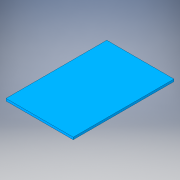
# Autodesk Inventor part: CBBLeft2
Saved by Autodesk Inventor 2019 (Build 230136000, 136)
## iProperties
Created: 2019-02-21
Part Number: CBBLeft2
Material: Generic
Document SubType Name: Modeling
Designer: james
Density: 1 g/cm^3
Appearance: Default(3)
Author: james
Autodesk Inventor part; units mm, degrees
ref_plane "YZ Plane" through (0, 0, 0) normal (1, 0, 0) x (0, 1, 0)
ref_plane "XZ Plane" through (0, 0, 0) normal (0, 1, 0) x (-1, 0, 0)
ref_plane "XY Plane" through (0, 0, 0) normal (0, 0, 1) x (1, 0, 0)
sketch "Sketch1" plane through (0, 0, 0) normal (0, 1, 0) x (-1, 0, 0)
  line L0 (59.2048, 125.73) -> (-93.1952, 125.73)
  line L1 (-93.1952, 125.73) -> (-93.1952, -102.87)
  line L2 (-93.1952, -102.87) -> (59.2048, -102.87)
  line L3 (59.2048, -102.87) -> (59.2048, 125.73)
  point P0 (0, 0)
  dimension "d0" = 228.6
  dimension "d1" = 152.4
  constraints: 8 end point, 2 parallel, 1 horizontal, 1 perpendicular
  measures "d0" distance of L2.end L0.start
  measures "d1" distance of L0.start L0.end
extrude "Extrusion1" add sketch "Sketch1" along normal blind 5.08
equation "\"d0\" = PartLength"
equation "\"d1\" = PartWidth"
equation "\"d2\" = WallWidth"
equation "\"DSLength\" = 1371.6"
equation "\"DSWidth\" = 304.8"
equation "\"DCDeckHeight\" = 76.2"
equation "\"WallWidth\" = 5.08"
equation "\"EdgeAngle\" = 10deg"
equation "\"LengthCuts\" = 152.4"
equation "\"WidthCuts\" = 50.8"
equation "\"PartLength\" = 228.6"
equation "\"PartWidth\" = 152.4"
equation "\"BoltHoldDiam\" = 6.35"
equation "\"ControlPlateLength\" = 228.6"
equation "\"ControlPlateWidth\" = 228.6"
equation "\"ControlPlateShelfLength\" = 19.05"
equation "\"ControlHoleLength\" = 190.5"
equation "\"ControlHoleWidth\" = 190.5"
equation "\"ControlHoleFromSide\" = 63.5"
equation "\"ControlHoleBoltHoleMid\" = 9.525"
equation "\"CPDeckHeight\" = 71.12"
equation "\"CPFromSide\" = 63.5"
equation "\"CPFromBack\" = 63.5"
equation "\"DU1CHWidth\" = 69.85"
equation "\"DU1CHLength\" = 146.05"
equation "\"ControlPlateScrewLength\" = 76.2"
equation "\"DSBackHeight\" = 127"
equation "\"BackShelf\" = 25.4"
equation "\"MainAngle\" = 168.22deg"
equation "\"CPDWidthHole\" = 120.65"
equation "\"CPDLengthHole\" = 146.05"
equation "\"DownBackHeight\" = 130.7084"
body "Solid1"
